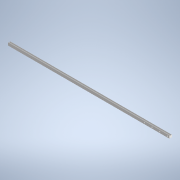
# Autodesk Inventor part: HSR30A128020 Rail
Saved by Autodesk Inventor 2022 (Build 260153000, 153)
## iProperties
Part Number: HSR30A128020 Rail
Material: Generic
Catalog Web Link: www.cadenas.de
Description: Flange Type - Heavy Load HSR-A Rail-
Vendor: THK
Document SubType Name: Modeling
Designer: partserver
Manufacturer: THK
Mass: 162.345 g
Surface Area: 356.21 cm^2
Volume: 162.345 cm^3
Density: 1 g/cm^3
Appearance: PSOLRGB-192-192-192
Category: PARTsolutions
Company: THK
NOB: 0
L: 0
GX: 0
LEND: 0
LMING: 0
LMAXG: 0
W1: 0
M1: 0
F: 0
D1: 0
D2: 0
HM: 0
MAXL: 0
H3: 0
ND: 0
GA: 0
X: 0
S1: 0
L1: 0
NOTE: 0
Title: HSR30A128020 Rail
Author: Cadenas PARTsolutions
Autodesk Inventor part; units mm, degrees
sketch "Sketch_17" plane through (-20, 0, 0) normal (1, 0, 0) x (0, 0, -1)
  line L0 (-14, 1.5) -> (-12.5, 0)
  line L1 (-12.5, 0) -> (-7.75, 0)
  line L2 (-7.75, 0) -> (-7.25, 0.5)
  line L3 (-7.25, 0.5) -> (-3.75, 0.5)
  line L4 (-3.75, 0.5) -> (-3.25, 0)
  line L5 (-3.25, 0) -> (3.25, 0)
  line L6 (3.25, 0) -> (3.75, 0.5)
  line L7 (3.75, 0.5) -> (7.25, 0.5)
  line L8 (7.25, 0.5) -> (7.75, 0)
  line L9 (7.75, 0) -> (12.5, 0)
  line L10 (12.5, 0) -> (14, 1.5)
  line L11 (14, 1.5) -> (14, 6.3)
  line L12 (14, 6.3) -> (9.3003, 10.9996)
  line L13 (9.3003, 10.9996) -> (9.3003, 15.0794)
  line L14 (9.3003, 15.0794) -> (10.9996, 16.7787)
  arc A0 (13.5309, 19.31) -> (10.9996, 16.7787) centre (13.8696, 16.4399) ccw
  line L15 (13.5309, 19.31) -> (14, 19.7791)
  line L16 (14, 19.7791) -> (14, 22.215)
  line L17 (14, 22.215) -> (13.5245, 22.6905)
  arc A1 (11.0003, 25.2147) -> (13.5245, 22.6905) centre (13.8696, 25.5598) ccw
  line L18 (11.0003, 25.2147) -> (10.215, 26)
  line L19 (10.215, 26) -> (-10.215, 26)
  line L20 (-10.215, 26) -> (-11.0003, 25.2147)
  arc A2 (-13.5245, 22.6905) -> (-11.0003, 25.2147) centre (-13.8696, 25.5598) ccw
  line L21 (-13.5245, 22.6905) -> (-14, 22.215)
  line L22 (-14, 22.215) -> (-14, 19.7791)
  line L23 (-14, 19.7791) -> (-13.5309, 19.31)
  arc A3 (-10.9996, 16.7787) -> (-13.5309, 19.31) centre (-13.8696, 16.4399) ccw
  line L24 (-10.9996, 16.7787) -> (-9.3003, 15.0794)
  line L25 (-9.3003, 15.0794) -> (-9.3003, 10.9996)
  line L26 (-9.3003, 10.9996) -> (-14, 6.3)
  line L27 (-14, 6.3) -> (-14, 1.5)
  constraints: 56 end point, 8 point on circle, 4 centre point
extrude "Extrusion1" add sketch "Sketch_17" along normal blind 1828.8
sketch "Sketch2" plane through (-20, 26, 10.215) normal (0, 1, 0) x (1, 0, 0)
  point P0 (20, 10.215)
hole "Hole1" at (0, 26, 0) direction (0, -1, 0) diameter 9 depth 26 counterbore diameter 14 counterbore depth 12
pattern_linear "Rectangular Pattern1" count 4 spacing 80 along (1, 0, 0) of "Hole1"
ref_plane "4dummy_XY" through (0, 0, 0) normal (1, 0, 0) x (0, 0, -1)
ref_plane "4dummy_YZ" through (0, 0, 0) normal (0, 0, -1) x (0, 1, 0)
ref_plane "4dummy_ZX" through (0, 0, 0) normal (0, 1, 0) x (1, 0, 0)
ref_plane "4slide_XY" through (-20, 7, 0) normal (1, 0, 0) x (0, 0, -1)
ref_plane "4slide_YZ" through (-20, 7, 0) normal (0, 0, -1) x (0, 1, 0)
ref_plane "4slide_ZX" through (-20, 7, 0) normal (0, 1, 0) x (1, 0, 0)
ref_plane "4track_XY" through (0, 0, 0) normal (0, 0, 1) x (1, 0, 0)
ref_plane "4track_YZ" through (0, 0, 0) normal (1, 0, 0) x (0, 1, 0)
ref_plane "4track_ZX" through (0, 0, 0) normal (0, 1, 0) x (0, 0, 1)
body "Solid1"
